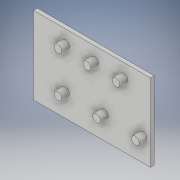
# Autodesk Inventor part: Backdrop base
Saved by Autodesk Inventor 2018 (Build 220112000, 112)
## iProperties
Created: 2018-12-13
Part Number: Backdrop base
Material: Generic
Document SubType Name: Modeling
Designer: F8PLTW
Density: 1 g/cm^3
Appearance: Default
Author: F8PLTW
Autodesk Inventor part; units mm, degrees
ref_plane "YZ Plane" through (0, 0, 0) normal (1, 0, 0) x (0, 1, 0)
ref_plane "XZ Plane" through (0, 0, 0) normal (0, 1, 0) x (-1, 0, 0)
ref_plane "XY Plane" through (0, 0, 0) normal (0, 0, 1) x (1, 0, 0)
sketch "Sketch1" plane through (0, 0, 0) normal (0, 0, 1) x (1, 0, 0)
  line L0 (-14.3848, 7.3422) -> (87.2152, 7.3422)
  line L1 (87.2152, 7.3422) -> (87.2152, -43.4578)
  line L2 (87.2152, -43.4578) -> (-14.3848, -43.4578)
  line L3 (-14.3848, -43.4578) -> (-14.3848, 7.3422)
  point P0 (0, 0)
  dimension "d0" = 101.6
  dimension "d1" = 50.8
  constraints: 8 end point, 2 parallel, 1 horizontal, 1 perpendicular
  measures "d0" distance of L1.end L2.end
  measures "d1" distance of L0.end L1.end
extrude "Extrusion1" add sketch "Sketch1" along normal blind 2.54
sketch "Sketch2" plane through (0, 0, 2.54) normal (0, 0, 1) x (1, 0, 0)
  circle A0 centre (6.7139, -1.3468) radius 2.54
  line L0 (6.7139, -1.3468) -> (25.7639, -1.3468) construction
  circle A1 centre (25.7639, -1.3468) radius 2.54
  line L1 (25.7639, -1.3468) -> (44.8139, -1.3468) construction
  circle A2 centre (44.8139, -1.3468) radius 2.54
  line L2 (-14.3848, 7.3422) -> (-14.3848, -43.4578) projected
  line L3 (-14.3848, -18.0578) -> (87.2152, -18.0578) construction
  line L4 (87.2152, -43.4578) -> (87.2152, 7.3422) projected
  circle A3 centre (6.7139, -28.1707) radius 2.54
  line L5 (6.7139, -28.1707) -> (32.1139, -28.1707) construction
  circle A4 centre (32.1139, -28.1707) radius 2.54
  line L6 (32.1139, -28.1707) -> (57.5139, -28.1707) construction
  circle A5 centre (57.5139, -28.1707) radius 2.54
  point P0 (0, 0)
  dimension "d4" = 5.08
  dimension "d5" = 19.05
  dimension "d6" = 5.08
  dimension "d7" = 19.05
  dimension "d8" = 5.08
  dimension "d9" = 5.08
  dimension "d10" = 25.4
  dimension "d11" = 5.08
  dimension "d12" = 25.4
  dimension "d13" = 5.08
  constraints: 10 end point, 6 centre point, 4 coincident, 4 horizontal, 2 midpoint
  measures "d4" diameter of A0
  measures "d5" distance of L0.start L0.end
  measures "d6" diameter of A1
  measures "d7" distance of L1.start L1.end
  measures "d8" diameter of A2
  measures "d9" diameter of A3
  measures "d10" distance of L5.start L5.end
  measures "d11" diameter of A4
  measures "d12" distance of L6.start L6.end
  measures "d13" diameter of A5
extrude "Extrusion2" add sketch "Sketch2" along normal blind 5.08
sketch "Sketch3" plane through (0, 0, 2.54) normal (0, 0, 1) x (1, 0, 0)
  line L0 (87.2152, -43.4578) -> (87.2152, 7.3422) projected
  line L1 (-14.3848, -43.4578) -> (87.2152, -43.4578) projected
  line L2 (87.2152, 7.3422) -> (62.3485, 7.3422)
  line L3 (62.3485, 7.3422) -> (62.3485, -43.4578)
  line L4 (62.3485, -43.4578) -> (87.2152, -43.4578)
  line L5 (87.2152, -43.4578) -> (87.2152, 7.3422)
  point P0 (0, 0)
  constraints: 8 end point, 2 parallel, 1 horizontal, 1 perpendicular, 1 point on line
extrude "Extrusion3" cut sketch "Sketch3" against normal blind 5.08
body "Solid1"
